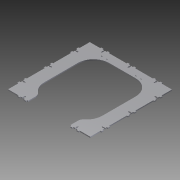
# Autodesk Inventor part: sostre
Saved by Autodesk Inventor 2012 (Build 160160000, 160)
## iProperties
Created: 2014-12-15
Part Number: sostre
Material: Default
Document SubType Name: Modeling
Designer: PRINCIPAL
Density: 1 g/cm^3
Author: PRINCIPAL
Autodesk Inventor part; units mm, degrees
ref_plane "YZ Plane" through (0, 0, 0) normal (1, 0, 0) x (0, 1, 0)
ref_plane "XZ Plane" through (0, 0, 0) normal (0, 1, 0) x (-1, 0, 0)
ref_plane "XY Plane" through (0, 0, 0) normal (0, 0, 1) x (1, 0, 0)
sketch "Boceto1" plane through (0, 0, 0) normal (0, 0, 1) x (1, 0, 0)
  arc A0 (-126.9286, -31.55) -> (-126.9286, -28.45) centre (-126.9286, -30) ccw
  line L0 (-126.9286, -31.55) -> (-130.4714, -31.55)
  arc A1 (-130.4714, -28.45) -> (-130.4714, -31.55) centre (-130.4714, -30) ccw
  line L1 (-130.4714, -28.45) -> (-126.9286, -28.45)
  arc A2 (-101.9286, -31.55) -> (-101.9286, -28.45) centre (-101.9286, -30) ccw
  line L2 (-101.9286, -31.55) -> (-105.4714, -31.55)
  arc A3 (-105.4714, -28.45) -> (-105.4714, -31.55) centre (-105.4714, -30) ccw
  line L3 (-105.4714, -28.45) -> (-101.9286, -28.45)
  line L4 (31.5286, -28.45) -> (35.0714, -28.45)
  arc A4 (35.0714, -31.55) -> (35.0714, -28.45) centre (35.0714, -30) ccw
  line L5 (35.0714, -31.55) -> (31.5286, -31.55)
  arc A5 (31.5286, -28.45) -> (31.5286, -31.55) centre (31.5286, -30) ccw
  line L6 (56.5286, -28.45) -> (60.0714, -28.45)
  arc A6 (60.0714, -31.55) -> (60.0714, -28.45) centre (60.0714, -30) ccw
  line L7 (60.0714, -31.55) -> (56.5286, -31.55)
  arc A7 (56.5286, -28.45) -> (56.5286, -31.55) centre (56.5286, -30) ccw
  line L8 (-120.2, -387.95) -> (-125.05, -387.95)
  line L9 (-125.05, -387.95) -> (-125.05, -392.95)
  line L10 (-125.05, -392.95) -> (-135.35, -392.95)
  line L11 (-135.35, -392.95) -> (-135.35, -387.95)
  line L12 (-135.35, -387.95) -> (-143.1167, -387.95)
  line L13 (-143.1167, -387.95) -> (-143.1167, -382.05)
  line L14 (-143.1167, -382.05) -> (-141.8667, -382.05)
  line L15 (-141.8667, -382.05) -> (-141.8667, -379.0834)
  line L16 (-141.8667, -379.0834) -> (-143.1167, -379.0834)
  line L17 (-143.1167, -379.0834) -> (-143.1167, -374.7834)
  line L18 (-143.1167, -374.7834) -> (-147.2833, -374.7834)
  line L19 (-147.2833, -374.7834) -> (-147.2833, -379.0834)
  line L20 (-147.2833, -379.0834) -> (-148.5333, -379.0834)
  line L21 (-148.5333, -379.0834) -> (-148.5333, -382.05)
  line L22 (-148.5333, -382.05) -> (-147.2833, -382.05)
  line L23 (-147.2833, -382.05) -> (-147.2833, -387.95)
  line L24 (-147.2833, -387.95) -> (-155.05, -387.95)
  line L25 (-155.05, -387.95) -> (-155.05, -392.95)
  line L26 (-155.05, -392.95) -> (-165.35, -392.95)
  line L27 (-165.35, -392.95) -> (-165.35, -387.95)
  line L28 (-165.35, -387.95) -> (-215.15, -387.95)
  line L29 (-215.15, -387.95) -> (-215.15, -339.15)
  line L30 (-215.15, -339.15) -> (-220.15, -339.15)
  line L31 (-220.15, -339.15) -> (-220.15, -328.85)
  line L32 (-220.15, -328.85) -> (-215.15, -328.85)
  line L33 (-215.15, -328.85) -> (-215.15, -321.0166)
  line L34 (-215.15, -321.0166) -> (-209.25, -321.0166)
  line L35 (-209.25, -321.0166) -> (-209.25, -322.2666)
  line L36 (-209.25, -322.2666) -> (-206.206, -322.2666)
  line L37 (-206.206, -322.2666) -> (-206.206, -321.0166)
  line L38 (-206.206, -321.0166) -> (-201.906, -321.0166)
  line L39 (-201.906, -321.0166) -> (-201.906, -316.8367)
  line L40 (-201.906, -316.8367) -> (-206.206, -316.8367)
  line L41 (-206.206, -316.8367) -> (-206.206, -315.5867)
  line L42 (-206.206, -315.5867) -> (-209.25, -315.5867)
  line L43 (-209.25, -315.5867) -> (-209.25, -316.8367)
  line L44 (-209.25, -316.8367) -> (-215.15, -316.8367)
  line L45 (-215.15, -316.8367) -> (-215.15, -309.15)
  line L46 (-215.15, -309.15) -> (-220.15, -309.15)
  line L47 (-220.15, -309.15) -> (-220.15, -298.85)
  line L48 (-220.15, -298.85) -> (-215.15, -298.85)
  line L49 (-215.15, -298.85) -> (-215.15, -214.15)
  line L50 (-215.15, -214.15) -> (-220.15, -214.15)
  line L51 (-220.15, -214.15) -> (-220.15, -203.85)
  line L52 (-220.15, -203.85) -> (-215.15, -203.85)
  line L53 (-215.15, -203.85) -> (-215.15, -196.0166)
  line L54 (-215.15, -196.0166) -> (-209.25, -196.0166)
  line L55 (-209.25, -196.0166) -> (-209.25, -197.2666)
  line L56 (-209.25, -197.2666) -> (-206.206, -197.2666)
  line L57 (-206.206, -197.2666) -> (-206.206, -196.0166)
  line L58 (-206.206, -196.0166) -> (-201.906, -196.0166)
  line L59 (-201.906, -196.0166) -> (-201.906, -191.8367)
  line L60 (-201.906, -191.8367) -> (-206.206, -191.8367)
  line L61 (-206.206, -191.8367) -> (-206.206, -190.5867)
  line L62 (-206.206, -190.5867) -> (-209.25, -190.5867)
  line L63 (-209.25, -190.5867) -> (-209.25, -191.8367)
  line L64 (-209.25, -191.8367) -> (-215.15, -191.8367)
  line L65 (-215.15, -191.8367) -> (-215.15, -184.15)
  line L66 (-215.15, -184.15) -> (-220.15, -184.15)
  line L67 (-220.15, -184.15) -> (-220.15, -173.85)
  line L68 (-220.15, -173.85) -> (-215.15, -173.85)
  line L69 (-215.15, -173.85) -> (-215.15, -89.15)
  line L70 (-215.15, -89.15) -> (-220.15, -89.15)
  line L71 (-220.15, -89.15) -> (-220.15, -78.85)
  line L72 (-220.15, -78.85) -> (-215.15, -78.85)
  line L73 (-215.15, -78.85) -> (-215.15, -71.0166)
  line L74 (-215.15, -71.0166) -> (-209.25, -71.0166)
  line L75 (-209.25, -71.0166) -> (-209.25, -72.2666)
  line L76 (-209.25, -72.2666) -> (-206.206, -72.2666)
  line L77 (-206.206, -72.2666) -> (-206.206, -71.0166)
  line L78 (-206.206, -71.0166) -> (-201.906, -71.0166)
  line L79 (-201.906, -71.0166) -> (-201.906, -66.8367)
  line L80 (-201.906, -66.8367) -> (-206.206, -66.8367)
  line L81 (-206.206, -66.8367) -> (-206.206, -65.5867)
  line L82 (-206.206, -65.5867) -> (-209.25, -65.5867)
  line L83 (-209.25, -65.5867) -> (-209.25, -66.8367)
  line L84 (-209.25, -66.8367) -> (-215.15, -66.8367)
  line L85 (-215.15, -66.8367) -> (-215.15, -59.15)
  line L86 (-215.15, -59.15) -> (-220.15, -59.15)
  line L87 (-220.15, -59.15) -> (-220.15, -48.85)
  line L88 (-220.15, -48.85) -> (-215.15, -48.85)
  line L89 (-215.15, -48.85) -> (-215.15, -0.05)
  line L90 (-215.15, -0.05) -> (-165.35, -0.05)
  line L91 (-165.35, -0.05) -> (-165.35, 4.95)
  line L92 (-165.35, 4.95) -> (-155.05, 4.95)
  line L93 (-155.05, 4.95) -> (-155.05, -0.05)
  line L94 (-155.05, -0.05) -> (-147.2833, -0.05)
  line L95 (-147.2833, -0.05) -> (-147.2833, -5.95)
  line L96 (-147.2833, -5.95) -> (-148.5333, -5.95)
  line L97 (-148.5333, -5.95) -> (-148.5333, -8.9833)
  line L98 (-148.5333, -8.9833) -> (-147.2833, -8.9833)
  line L99 (-147.2833, -8.9833) -> (-147.2833, -14.6327)
  line L100 (-147.2833, -14.6327) -> (-143.1167, -14.6327)
  line L101 (-143.1167, -14.6327) -> (-143.1167, -8.9833)
  line L102 (-143.1167, -8.9833) -> (-141.8667, -8.9833)
  line L103 (-141.8667, -8.9833) -> (-141.8667, -5.95)
  line L104 (-141.8667, -5.95) -> (-143.1167, -5.95)
  line L105 (-143.1167, -5.95) -> (-143.1167, -0.05)
  line L106 (-143.1167, -0.05) -> (-135.35, -0.05)
  line L107 (-135.35, -0.05) -> (-135.35, 4.95)
  line L108 (-135.35, 4.95) -> (-125.05, 4.95)
  line L109 (-125.05, 4.95) -> (-125.05, -0.05)
  line L110 (-125.05, -0.05) -> (-40.35, -0.05)
  line L111 (-40.35, -0.05) -> (-40.35, 4.95)
  line L112 (-40.35, 4.95) -> (-30.05, 4.95)
  line L113 (-30.05, 4.95) -> (-30.05, -0.05)
  line L114 (-30.05, -0.05) -> (-22.2833, -0.05)
  line L115 (-22.2833, -0.05) -> (-22.2833, -5.95)
  line L116 (-22.2833, -5.95) -> (-23.5333, -5.95)
  line L117 (-23.5333, -5.95) -> (-23.5333, -8.9833)
  line L118 (-23.5333, -8.9833) -> (-22.2833, -8.9833)
  line L119 (-22.2833, -8.9833) -> (-22.2833, -14.6327)
  line L120 (-22.2833, -14.6327) -> (-18.1167, -14.6327)
  line L121 (-18.1167, -14.6327) -> (-18.1167, -8.9833)
  line L122 (-18.1167, -8.9833) -> (-16.8667, -8.9833)
  line L123 (-16.8667, -8.9833) -> (-16.8667, -5.95)
  line L124 (-16.8667, -5.95) -> (-18.1167, -5.95)
  line L125 (-18.1167, -5.95) -> (-18.1167, -0.05)
  line L126 (-18.1167, -0.05) -> (-10.35, -0.05)
  line L127 (-10.35, -0.05) -> (-10.35, 4.95)
  line L128 (-10.35, 4.95) -> (-0.05, 4.95)
  line L129 (-0.05, 4.95) -> (-0.05, -0.05)
  line L130 (-0.05, -0.05) -> (84.65, -0.05)
  line L131 (84.65, -0.05) -> (84.65, 4.95)
  line L132 (84.65, 4.95) -> (94.95, 4.95)
  line L133 (94.95, 4.95) -> (94.95, -0.05)
  line L134 (94.95, -0.05) -> (102.7167, -0.05)
  line L135 (102.7167, -0.05) -> (102.7167, -5.95)
  line L136 (102.7167, -5.95) -> (101.4667, -5.95)
  line L137 (101.4667, -5.95) -> (101.4667, -8.9833)
  line L138 (101.4667, -8.9833) -> (102.7167, -8.9833)
  line L139 (102.7167, -8.9833) -> (102.7167, -14.6327)
  line L140 (102.7167, -14.6327) -> (106.8833, -14.6327)
  line L141 (106.8833, -14.6327) -> (106.8833, -8.9833)
  line L142 (106.8833, -8.9833) -> (108.1333, -8.9833)
  line L143 (108.1333, -8.9833) -> (108.1333, -5.95)
  line L144 (108.1333, -5.95) -> (106.8833, -5.95)
  line L145 (106.8833, -5.95) -> (106.8833, -0.05)
  line L146 (106.8833, -0.05) -> (114.65, -0.05)
  line L147 (114.65, -0.05) -> (114.65, 4.95)
  line L148 (114.65, 4.95) -> (124.95, 4.95)
  line L149 (124.95, 4.95) -> (124.95, -0.05)
  line L150 (124.95, -0.05) -> (174.75, -0.05)
  line L151 (174.75, -0.05) -> (174.75, -48.85)
  line L152 (174.75, -48.85) -> (179.75, -48.85)
  line L153 (179.75, -48.85) -> (179.75, -59.15)
  line L154 (179.75, -59.15) -> (174.75, -59.15)
  line L155 (174.75, -59.15) -> (174.75, -66.8367)
  line L156 (174.75, -66.8367) -> (168.85, -66.8367)
  line L157 (168.85, -66.8367) -> (168.85, -65.5867)
  line L158 (168.85, -65.5867) -> (165.8167, -65.5867)
  line L159 (165.8167, -65.5867) -> (165.8167, -66.8367)
  line L160 (165.8167, -66.8367) -> (161.5167, -66.8367)
  line L161 (161.5167, -66.8367) -> (161.5167, -71.0166)
  line L162 (161.5167, -71.0166) -> (165.8167, -71.0166)
  line L163 (165.8167, -71.0166) -> (165.8167, -72.2666)
  line L164 (165.8167, -72.2666) -> (168.85, -72.2666)
  line L165 (168.85, -72.2666) -> (168.85, -71.6416)
  line L166 (168.85, -71.6416) -> (168.85, -71.0166)
  line L167 (168.85, -71.0166) -> (174.75, -71.0166)
  line L168 (174.75, -71.0166) -> (174.75, -78.85)
  line L169 (174.75, -78.85) -> (179.75, -78.85)
  line L170 (179.75, -78.85) -> (179.75, -89.15)
  line L171 (179.75, -89.15) -> (174.75, -89.15)
  line L172 (174.75, -89.15) -> (174.75, -173.85)
  line L173 (174.75, -173.85) -> (179.75, -173.85)
  line L174 (179.75, -173.85) -> (179.75, -184.15)
  line L175 (179.75, -184.15) -> (174.75, -184.15)
  line L176 (174.75, -184.15) -> (174.75, -191.8367)
  line L177 (174.75, -191.8367) -> (168.85, -191.8367)
  line L178 (168.85, -191.8367) -> (168.85, -190.5867)
  line L179 (168.85, -190.5867) -> (165.8167, -190.5867)
  line L180 (165.8167, -190.5867) -> (165.8167, -191.8367)
  line L181 (165.8167, -191.8367) -> (161.5167, -191.8367)
  line L182 (161.5167, -191.8367) -> (161.5167, -196.0166)
  line L183 (161.5167, -196.0166) -> (165.8167, -196.0166)
  line L184 (165.8167, -196.0166) -> (165.8167, -197.2666)
  line L185 (165.8167, -197.2666) -> (168.85, -197.2666)
  line L186 (168.85, -197.2666) -> (168.85, -196.0166)
  line L187 (168.85, -196.0166) -> (174.75, -196.0166)
  line L188 (174.75, -196.0166) -> (174.75, -203.85)
  line L189 (174.75, -203.85) -> (179.75, -203.85)
  line L190 (179.75, -203.85) -> (179.75, -214.15)
  line L191 (179.75, -214.15) -> (174.75, -214.15)
  line L192 (174.75, -214.15) -> (174.75, -298.85)
  line L193 (174.75, -298.85) -> (179.75, -298.85)
  line L194 (179.75, -298.85) -> (179.75, -309.15)
  line L195 (179.75, -309.15) -> (174.75, -309.15)
  line L196 (174.75, -309.15) -> (174.75, -316.8367)
  line L197 (174.75, -316.8367) -> (168.85, -316.8367)
  line L198 (168.85, -316.8367) -> (168.85, -315.5867)
  line L199 (168.85, -315.5867) -> (165.8167, -315.5867)
  line L200 (165.8167, -315.5867) -> (165.8167, -316.8367)
  line L201 (165.8167, -316.8367) -> (161.5167, -316.8367)
  line L202 (161.5167, -316.8367) -> (161.5167, -321.0166)
  line L203 (161.5167, -321.0166) -> (165.8167, -321.0166)
  line L204 (165.8167, -321.0166) -> (165.8167, -322.2666)
  line L205 (165.8167, -322.2666) -> (168.85, -322.2666)
  line L206 (168.85, -322.2666) -> (168.85, -321.0166)
  line L207 (168.85, -321.0166) -> (174.75, -321.0166)
  line L208 (174.75, -321.0166) -> (174.75, -328.85)
  line L209 (174.75, -328.85) -> (179.75, -328.85)
  line L210 (179.75, -328.85) -> (179.75, -339.15)
  line L211 (179.75, -339.15) -> (174.75, -339.15)
  line L212 (174.75, -339.15) -> (174.75, -387.95)
  line L213 (174.75, -387.95) -> (124.95, -387.95)
  line L214 (124.95, -387.95) -> (124.95, -392.95)
  line L215 (124.95, -392.95) -> (114.65, -392.95)
  line L216 (114.65, -392.95) -> (114.65, -387.95)
  line L217 (114.65, -387.95) -> (106.8833, -387.95)
  line L218 (106.8833, -387.95) -> (106.8833, -382.05)
  line L219 (106.8833, -382.05) -> (108.1333, -382.05)
  line L220 (108.1333, -382.05) -> (108.1333, -379.0834)
  line L221 (108.1333, -379.0834) -> (106.8833, -379.0834)
  line L222 (106.8833, -379.0834) -> (106.8833, -374.7834)
  line L223 (106.8833, -374.7834) -> (102.7167, -374.7834)
  line L224 (102.7167, -374.7834) -> (102.7167, -379.0834)
  line L225 (102.7167, -379.0834) -> (101.4667, -379.0834)
  line L226 (101.4667, -379.0834) -> (101.4667, -382.05)
  line L227 (101.4667, -382.05) -> (102.7167, -382.05)
  line L228 (102.7167, -382.05) -> (102.7167, -387.95)
  line L229 (102.7167, -387.95) -> (94.95, -387.95)
  line L230 (94.95, -387.95) -> (94.95, -392.95)
  line L231 (94.95, -392.95) -> (84.65, -392.95)
  line L232 (84.65, -392.95) -> (84.65, -387.95)
  line L233 (84.65, -387.95) -> (79.8, -387.95)
  line L234 (79.8, -387.95) -> (79.8, -351.0625)
  arc A8 (89.175, -331.5468) -> (79.8, -351.0625) centre (104.8, -351.0625) ccw
  arc A9 (89.175, -331.5468) -> (117.3, -273) centre (42.3, -273) ccw
  line L235 (117.3, -273) -> (117.3, -115)
  arc A10 (117.3, -115) -> (42.3, -40) centre (42.3, -115) ccw
  line L236 (42.3, -40) -> (-82.7, -40)
  arc A11 (-82.7, -40) -> (-157.7, -115) centre (-82.7, -115) ccw
  line L237 (-157.7, -115) -> (-157.7, -273)
  arc A12 (-157.7, -273) -> (-129.575, -331.5468) centre (-82.7, -273) ccw
  arc A13 (-120.2, -351.0625) -> (-129.575, -331.5468) centre (-145.2, -351.0625) ccw
  line L238 (-120.2, -351.0625) -> (-120.2, -387.95)
  point P0 (0, 0)
  dimension "d2" = 21.4571
  dimension "d3" = 21.4571
  dimension "d6" = 0
  dimension "d7" = 162
  constraints: 478 end point, 28 point on circle, 14 centre point
  measures "d2" distance of A3.centre A0.centre
  measures "d3" distance of A4.centre A7.centre
  measures "d6" distance of point (-130.471, -30) A1.centre
  measures "d7" distance of A5.centre A1.centre
extrude "Extrusión1" add sketch "Boceto1" along normal blind 5
